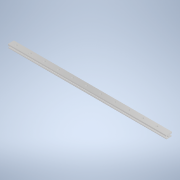
# Autodesk Inventor part: Fuehrungsschiene440mm
Saved by Autodesk Inventor 2021.3 (Build 253353000, 353)
## iProperties
Created: 2021-04-14
Part Number: Fuehrungsschiene440mm
Material: Generic
Document SubType Name: Modeling
Designer: Fabijan_Sven
Density: 1 g/cm^3
Appearance: Aluminum - Dark
Author: Fabijan_Sven
Autodesk Inventor part; units mm, degrees
ref_plane "YZ Plane" through (0, 0, 0) normal (1, 0, 0) x (0, 1, 0)
ref_plane "XZ Plane" through (0, 0, 0) normal (0, 1, 0) x (-1, 0, 0)
ref_plane "XY Plane" through (0, 0, 0) normal (0, 0, 1) x (1, 0, 0)
sketch "Sketch1" plane through (0, 0, 0) normal (1, 0, 0) x (0, 1, 0)
  line L0 (10.8, 8.5) -> (7, 8.5)
  line L1 (7, -8.5) -> (10.8, -8.5)
  line L2 (10.8, -8.5) -> (10.8, 8.5)
  line L3 (1.8, 7.5) -> (0, 7.5)
  line L4 (0, 7.5) -> (0, -7.5)
  line L5 (0, -7.5) -> (1.8, -7.5)
  line L6 (7, 8.5) -> (7, 4.25)
  line L7 (1.8, -7.5) -> (1.8, -4.25)
  arc A0 (5, 2.25) -> (7, 4.25) centre (5, 4.25) ccw
  arc A1 (7, -4.25) -> (5, -2.25) centre (5, -4.25) ccw
  arc A2 (3.8, -2.25) -> (1.8, -4.25) centre (3.8, -4.25) ccw
  arc A3 (1.8, 4.25) -> (3.8, 2.25) centre (3.8, 4.25) ccw
  line L8 (5, 2.25) -> (3.8, 2.25)
  line L9 (1.8, 4.25) -> (1.8, 7.5)
  line L10 (3.8, -2.25) -> (5, -2.25)
  line L11 (7, -4.25) -> (7, -8.5)
  point P0 (0, 0)
  dimension "d0" = 17
  dimension "d1" = 15
  dimension "d2" = 10.8
  dimension "d4" = 1.8
  dimension "d6" = 8.5
  dimension "d8" = 7.5
  dimension "d9" = 0
  dimension "d19" = 2
  dimension "d20" = 2
  dimension "d21" = 4.25
  dimension "d23" = 7
  dimension "d24" = 2
  dimension "d25" = 4.25
  dimension "d28" = 2
  dimension "d29" = 2
  dimension "d31" = 2
  dimension "d32" = 2
  dimension "d33" = 2
  dimension "d34" = 2
  dimension "d35" = 2
  constraints: 25 end point, 11 point on circle, 7 parallel, 4 centre point, 3 horizontal, 3 perpendicular, 2 collinear, 2 point on line, 2 tangent
  measures "d0" distance of L1.end L0.start
  measures "d1" distance of L3.end L4.end
  measures "d2" distance between parallel lines of L2 L4
  measures "d4" distance between parallel lines of L7 L4
  measures "d6" distance from line of L0 point (0, 0)
  measures "d8" distance from line of point (0, 0) L3
  measures "d9" distance from line of point (0, 0) L4
  measures "d19" distance from line of L8.start L6
  measures "d20" distance from line of L8 L6.end
  measures "d21" distance from line of L0 L6.end
  measures "d23" distance between parallel lines of L4 L11
  measures "d24" distance from line of L10 L11.start
  measures "d25" distance from line of L1 L11.start
  measures "d28" distance from line of L9 L8.end
  measures "d29" distance from line of L8 L9.start
  measures "d31" distance from line of L7 A2.centre
  measures "d32" distance from line of A2.end L10
  measures "d33" distance from line of L11 L10.end
  measures "d34" distance from line of A1.centre L11
  measures "d35" distance from line of A2.centre L10
extrude "Schiene" add sketch "Sketch1" along normal blind 450
sketch "Sketch2" plane through (0, 10.8, 8.5) normal (0, 1, 0) x (1, 0, 0)
  circle A0 centre (95, 8.5) radius 1.5
  circle A1 centre (55, 8.5) radius 1.5
  circle A2 centre (15, 8.5) radius 1.5
  circle A3 centre (135, 8.5) radius 1.5
  circle A4 centre (175, 8.5) radius 1.5
  circle A5 centre (215, 8.5) radius 1.5
  circle A6 centre (255, 8.5) radius 1.5
  circle A7 centre (295, 8.5) radius 1.5
  line L0 (0, 8.5) -> (450, 8.5) construction
  line L1 (450, 17) -> (450, 0) projected
  line L2 (0, 17) -> (0, 0) projected
  circle A8 centre (335, 8.5) radius 1.5
  circle A9 centre (375, 8.5) radius 1.5
  circle A10 centre (415, 8.5) radius 1.5
  line L3 (-48.7314, 8.5) -> (450.9636, 8.5) construction
  dimension "d38" = 15
  dimension "d39" = 40
  dimension "d40" = 40
  dimension "d41" = 40
  dimension "d42" = 40
  dimension "d43" = 40
  dimension "d44" = 40
  dimension "d48" = 40
  dimension "d49" = 40
  dimension "d53" = 40
  dimension "d54" = 40
  dimension "d59" = 3
  dimension "d60" = 3
  dimension "d61" = 3
  dimension "d62" = 3
  dimension "d63" = 3
  dimension "d64" = 3
  dimension "d65" = 3
  dimension "d66" = 3
  dimension "d67" = 3
  dimension "d68" = 3
  dimension "d69" = 3
  constraints: 11 centre point, 3 point on line, 2 end point, 1 midpoint, 12 other
  measures "d38" distance from line of A2.centre L2
  measures "d39" distance of A1.centre A2.centre
  measures "d40" distance of A1.centre A0.centre
  measures "d41" distance of A0.centre A3.centre
  measures "d42" distance of A3.centre A4.centre
  measures "d43" distance of A4.centre A5.centre
  measures "d44" distance of A5.centre A6.centre
  measures "d48" distance of A8.centre A9.centre
  measures "d49" distance of A9.centre A10.centre
  measures "d53" distance of A7.centre A6.centre
  measures "d54" distance of A8.centre A7.centre
  measures "d59" diameter of A10
  measures "d60" diameter of A9
  measures "d61" diameter of A8
  measures "d62" diameter of A7
  measures "d63" diameter of A6
  measures "d64" diameter of A5
  measures "d65" diameter of A4
  measures "d66" diameter of A3
  measures "d67" diameter of A0
  measures "d68" diameter of A1
  measures "d69" diameter of A2
hole "Hole1" at (415, 10.8, 0) at (375, 10.8, 0) at (335, 10.8, 0) at (295, 10.8, 0) at (255, 10.8, 0) at (215, 10.8, 0) at (175, 10.8, 0) at (135, 10.8, 0) at (95, 10.8, 0) at (55, 10.8, 0) at (15, 10.8, 0) direction (0, -1, 0) diameter 3 depth 20 tip angle 118 counterbore diameter 6 counterbore depth 3.5
equation "\"d93\" = d68"
body "Solid1"
